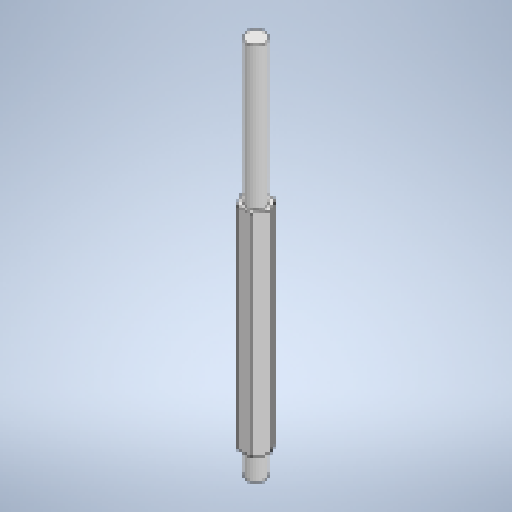
# Autodesk Inventor part: NVPH-201 shredder shaft
Saved by Autodesk Inventor 2025.1 (Build 291241020, 241B)
## iProperties
Created: 2024-12-04
Part Number: NVPH-201 shredder shaft
Material: Generic
Document SubType Name: Modeling
Designer: DELL
Density: 1 g/cm^3
Appearance: Default
Author: DELL
Autodesk Inventor part; units mm, degrees
ref_plane "YZ Plane" through (0, 0, 0) normal (1, 0, 0) x (0, 1, 0)
ref_plane "XZ Plane" through (0, 0, 0) normal (0, 1, 0) x (-1, 0, 0)
ref_plane "XY Plane" through (0, 0, 0) normal (0, 0, 1) x (1, 0, 0)
sketch "Sketch1" plane through (0, 0, 0) normal (0, 0, 1) x (1, 0, 0)
  line L0 (-11.547, -20) -> (-23.094, 0)
  line L1 (-23.094, 0) -> (-11.547, 20)
  line L2 (-11.547, 20) -> (11.547, 20)
  line L3 (11.547, 20) -> (23.094, 0)
  line L4 (23.094, 0) -> (11.547, -20)
  line L5 (11.547, -20) -> (-11.547, -20)
  point P0 (0, 0)
  point P1 (0, 0)
  dimension "d0" = 40
  constraints: 12 end point, 1 coincident, 1 horizontal, 13 other
  measures "d0" distance between parallel lines of L5 L2
extrude "Extrusion1" add sketch "Sketch1" along normal mid plane 340
sketch "Sketch3" plane through (0, 0, 0) normal (0, 1, 0) x (-1, 0, 0)
  line L0 (0, -230) -> (0, 0)
  line L1 (0, 0) -> (0, 400)
  line L2 (0, 400) -> (-14, 400)
  line L3 (-14, 400) -> (-14, 320)
  line L4 (-14, 320) -> (-15, 320)
  line L5 (-15, 320) -> (-15, 0)
  line L6 (-15, 0) -> (-15, -230)
  line L7 (-15, -230) -> (0, -230)
  dimension "d8" = 30
  dimension "d9" = 230
  dimension "d10" = 400
  dimension "d11" = 80
  dimension "d12" = 28
  constraints: 16 end point, 5 perpendicular, 2 point on line, 1 vertical
  measures "d8" diameter of L6 L0
  measures "d9" distance from line of L0.end L7
  measures "d10" distance of L1.end L0.end
  measures "d11" distance between parallel lines of L2 L4
  measures "d12" diameter of L3 L1
revolve "Revolution1" add sketch "Sketch3" angle 360 about axis through (0, 0, -230) along (0, 0, 1)
body "Solid1"
